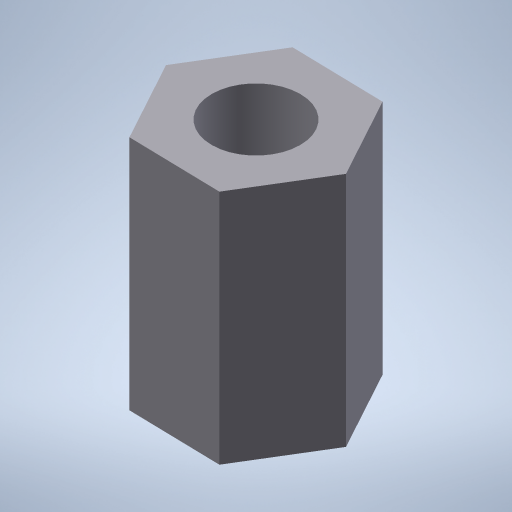
# Autodesk Inventor part: standoff815mm
Saved by Autodesk Inventor 2024 (Build 280153000, 153)
## iProperties
Created: 2011-03-09
Part Number: standoff815mm
Material: Aluminum-6061
Document SubType Name: Modeling
Designer: Robert Davis
Mass: 0.438627 g
Surface Area: 2.71685 cm^2
Volume: 0.161855 cm^3
Density: 2.71 g/cm^3
Description: AL SPACER
Appearance: Aluminum - Flat
Author: Robert Davis
Autodesk Inventor part; units mm, degrees
ref_plane "YZ Plane" through (0, 0, 0) normal (1, 0, 0) x (0, 1, 0)
ref_plane "XZ Plane" through (0, 0, 0) normal (0, 1, 0) x (-1, 0, 0)
ref_plane "XY Plane" through (0, 0, 0) normal (0, 0, 1) x (1, 0, 0)
sketch "Sketch1" plane through (0, 0, 0) normal (0, 0, 1) x (1, 0, 0)
  circle A0 centre (0, 0) radius 1.524
  line L0 (-1.524, 2.7853) -> (1.6502, 2.7125)
  line L1 (1.6502, 2.7125) -> (3.1742, -0.0728)
  line L2 (3.1742, -0.0728) -> (1.524, -2.7853)
  line L3 (1.524, -2.7853) -> (-1.6502, -2.7125)
  line L4 (-1.6502, -2.7125) -> (-3.1742, 0.0728)
  line L5 (-3.1742, 0.0728) -> (-1.524, 2.7853)
  dimension "d1" = 3.048
  constraints: 12 end point, 1 centre point, 13 other
  measures "d1" diameter of A0
extrude "Extrusion2" add sketch "Sketch1" along normal blind 8.15
body "Solid2"
